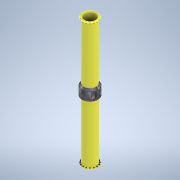
# Autodesk Inventor part: pipe_anode
Saved by Autodesk Inventor 2022 (Build 260153000, 153)
## iProperties
Created: 2021-12-16
Part Number: pipe_anode
Material: Steel
Document SubType Name: Modeling
Designer: jpc
Density: 7.85 g/cm^3
Appearance: Steel Galvanized
Mass: 2.14484e+06 g
Surface Area: 119776 cm^2
Volume: 273228 cm^3
Author: jpc
Autodesk Inventor part; units mm, degrees
ref_plane "XZ Plane" through (0, 0, 0) normal (0, 1, 0) x (-1, 0, 0)
ref_plane "XY Plane" through (0, 0, 0) normal (0, 0, 1) x (1, 0, 0)
sketch "cross_section" plane through (0, 0, 0) normal (0, 1, 0) x (-1, 0, 0)
  circle A0 centre (0, 0) radius 500
  circle A1 centre (0, 0) radius 450
  dimension "dia_out" = 1000
  dimension "dia_in" = 900
  constraints: 2 centre point, 2 coincident
  measures "dia_out" diameter of A0
  measures "dia_in" diameter of A1
sketch "curved_midline" plane through (0, 0, 0) normal (0, 0, 1) x (1, 0, 0)
  arc A0 (1000, 1000) -> (0, 0) centre (1000, 0) ccw
  line L0 (0, 0) -> (1000, 0) construction
  line L1 (1000, 0) -> (1000, 1000) construction
  dimension "d4" = 1000
  constraints: 4 end point, 2 point on circle, 1 centre point, 1 horizontal, 1 perpendicular
  measures "d4" distance of L0.end L1.end
sketch "straight_midline" plane through (0, 0, 0) normal (0, 0, 1) x (1, 0, 0)
  line L0 (0, 0) -> (0, 10000)
  dimension "len" = 10000
  constraints: 2 end point, 1 vertical
  measures "len" distance of L0.start L0.end
sweep "Sweep" add profiles "cross_section" path "straight_midline"
sketch "Sketch4" plane through (0, 0, 0) normal (0, -1, 0) x (1, 0, 0)
  circle A0 centre (0, 0) radius 600
  circle A1 centre (0, 0) radius 450 projected
  dimension "endcap_dia" = 1200
  constraints: 1 centre point, 1 coincident
  measures "endcap_dia" diameter of A0
extrude "Endcap" add sketch "Sketch4" against normal blind 50
ref_plane "Midplane" through (0, 5000, 0) normal (0, -1, 0) x (1, 0, 0)
chamfer "Chamfer" distance 12.5 angle 45 1 edges at (-600, 0, 0)
sketch "Sketch7" plane through (0, 50, 0) normal (0, 1, 0) x (1, 0, 0)
  circle A0 centre (0, 0) radius 600 construction
  circle A1 centre (0, 0) radius 600 construction
  line L0 (-600, 0) -> (-499.1664, 0) construction
  circle A2 centre (-549.5832, 0) radius 25.2084
  circle A3 centre (0, 0) radius 450 projected
  circle A4 centre (0, 0) radius 500 projected
  dimension "d27" = 100.8336
  dimension "d28" = 50.4168
  constraints: 2 end point, 1 centre point, 1 horizontal, 1 horizontal alignment, 1 midpoint, 1 other
  measures "d27" distance of L0.start L0.end
  measures "d28" diameter of A2
extrude "Hole" cut sketch "Sketch7" against normal through all contours A2
pattern_circular "Holes" count 16 over 360 about axis through (0, -10, 0) along (0, 1, 0) of "Hole"
mirror "MirroredFeatures" about plane through (0, 5000, 0) normal (0, -1, 0) of "Hole", "Holes", "Endcap", "Chamfer"
sketch "Sketch8" plane through (0, 50, 0) normal (0, 1, 0) x (1, 0, 0)
  circle A0 centre (-549.5832, 0) radius 25.2084 construction
  circle A1 centre (-549.5832, 0) radius 37.8126 construction
  circle A2 centre (0, 0) radius 587.5 construction
  line L0 (-587.5, 0) -> (-568.5416, 32.8369)
  line L1 (-568.5416, 32.8369) -> (-530.6248, 32.8369)
  line L2 (-530.6248, 32.8369) -> (-511.6664, 0)
  line L3 (-511.6664, 0) -> (-530.6248, -32.8369)
  line L4 (-530.6248, -32.8369) -> (-568.5416, -32.8369)
  line L5 (-568.5416, -32.8369) -> (-587.5, 0)
  dimension "d34" = 50.4168
  dimension "d35" = 75.6252
  constraints: 12 end point, 2 coincident, 1 centre point, 1 horizontal, 1 horizontal alignment, 14 other
  measures "d34" diameter of A0
  measures "d35" diameter of A1
extrude "BoltHead" add sketch "Sketch8" along normal blind 37.5 separate body
sketch "Sketch9" plane through (0, 50, 0) normal (0, -1, 0) x (1, 0, 0)
  circle A0 centre (-549.5832, 0) radius 25.2084 projected
  point P0 (0, 0)
extrude "BoltThreadHalf" add sketch "Sketch9" along normal blind 45 bodies 2
pattern_circular "BoltHalves" count 16 over 360 about axis through (0, -10, 0) along (0, 1, 0) bodies 2
mirror "MirroredBolts" about plane through (0, 5000, 0) normal (0, -1, 0) bodies 2
sketch "Sketch10" plane through (-530.6248, 9912.5, 32.8369) normal (0, -1, 0) x (0, 0, 1)
  circle A0 centre (-32.8369, 18.9584) radius 25.2084 projected
  point P0 (-32.8369, -530.6248)
extrude "ExtraThread" add sketch "Sketch10" along normal blind 22.5 bodies 2
chamfer "ThreadChamfer" distance 6.25 angle 45 1 edges at (-549.5832, 9890, -25.2084)
pattern_circular "Circular Pattern5" count 16 over 360 about axis through (0, 9950, 0) along (0, 1, 0) of "ExtraThread", "ThreadChamfer" bodies 2
sketch "Sketch11" plane through (0, 0, 0) normal (1, 0, 0) x (0, 1, 0)
  line L0 (10000, 450) -> (0, 450) construction
  line L1 (4491.6667, 450) -> (4666.6667, 625)
  line L2 (4666.6667, 625) -> (5333.3333, 625)
  line L3 (5333.3333, 625) -> (5508.3333, 450)
  line L4 (5508.3333, 450) -> (4491.6667, 450)
  line L5 (50, 500) -> (9950, 500) construction
  line L6 (-2000, 0) -> (12000, 0) projected
  point P0 (0, 0)
  point P1 (5000, 450)
  dimension "d54" = 666.6667
  dimension "d55" = 125
  dimension "d56" = 45
  constraints: 8 end point, 2 midpoint, 2 point on line, 1 collinear, 1 parallel, 1 perpendicular
  measures "d54" distance of L1.end L2.end
  measures "d55" distance between parallel lines of L2 L5
  measures "d56" angle of L0 L3
revolve "Attachment" add sketch "Sketch11" angle 360 about axis through (0, -10, 0) along (0, 1, 0) separate body
ref_plane "AnodeInnerPlane" through (450, 5000, 0) normal (1, 0, 0) x (0, 1, 0)
ref_plane "AnodOuterPlane" through (625, 5000, 0) normal (1, 0, 0) x (0, 1, 0)
ref_plane "NodeMidplane" through (537.5, 5000, 0) normal (1, 0, 0) x (0, 1, 0)
ref_plane "AnodeCutPlane" through (493.75, 5000, 0) normal (1, 0, 0) x (0, 1, 0)
split body "Split" result two bodies by plane through (0, 0, 0) normal (0, 0, 1) bodies 3 first body at (450.0712, 4830.5556, 19.6505)
sketch "Sketch13" plane through (0, 0, 0) normal (0, 1, 0) x (-1, 0, 0)
  line L0 (781.25, 15.625) -> (-781.25, 15.625)
  line L1 (-781.25, 15.625) -> (-781.25, -15.625)
  line L2 (-781.25, -15.625) -> (781.25, -15.625)
  line L3 (781.25, -15.625) -> (781.25, 15.625)
  arc A0 (-625, 0) -> (625, 0) centre (0, 0) ccw projected
  line L4 (625, 0) -> (450, 0) projected
  line L5 (781.25, 15.625) -> (-781.25, -15.625) construction
  dimension "d58" = 625
  dimension "d59" = 1562.5
  dimension "d60" = 31.25
  constraints: 10 end point, 2 parallel, 1 coincident, 1 horizontal, 1 midpoint, 1 perpendicular
  measures "d58" radius of A0
  measures "d59" distance of L1.end L2.end
  measures "d60" distance of L2.end L0.start
extrude "Separate" cut sketch "Sketch13" along normal through all both and the other way through all contours L3 L2 L1 L0 bodies 5 4
sketch "Sketch15" plane through (625, 5000, 0) normal (1, 0, 0) x (0, 1, 0)
  line L0 (-333.3333, 15.625) -> (333.3333, 15.625) construction
  line L1 (333.3333, 15.625) -> (333.3333, 15.625) construction
  line L2 (333.3333, 15.625) -> (-333.3333, 15.625) construction
  line L3 (-333.3333, 15.625) -> (-333.3333, 15.625) construction
  line L4 (333.3333, -15.625) -> (-333.3333, -15.625) construction
  line L5 (-333.3333, -15.625) -> (-333.3333, -15.625) construction
  line L6 (-333.3333, -15.625) -> (333.3333, -15.625) construction
  line L7 (333.3333, -15.625) -> (333.3333, -15.625) construction
  line L8 (333.3333, 15.625) -> (333.3333, 625) construction
  line L9 (-333.3333, 625) -> (333.3333, 625) construction
  line L10 (-333.3333, 15.625) -> (-333.3333, 625) construction
  line L11 (-333.3333, -625) -> (-333.3333, -15.625) construction
  line L12 (-333.3333, -625) -> (333.3333, -625) construction
  line L13 (333.3333, -625) -> (333.3333, -15.625) construction
  line L14 (250, 396.4844) -> (-250, 396.4844)
  line L15 (-250, 396.4844) -> (-250, 91.7969)
  line L16 (-250, 91.7969) -> (250, 91.7969)
  line L17 (250, 91.7969) -> (250, 396.4844)
  line L18 (250, -91.7969) -> (-250, -91.7969)
  line L19 (-250, -91.7969) -> (-250, -396.4844)
  line L20 (-250, -396.4844) -> (250, -396.4844)
  line L21 (250, -396.4844) -> (250, -91.7969)
  line L22 (0, 91.7969) -> (0, 15.625) construction
  point P0 (-5000, 0)
  dimension "d63" = 609.375
  dimension "d64" = 304.6875
  dimension "d65" = 666.6667
  dimension "d66" = 500
  dimension "d67" = 76.1719
  dimension "d68" = 76.1719
  constraints: 18 end point, 4 parallel, 3 perpendicular, 2 equal length, 2 horizontal, 2 midpoint, 1 collinear
  measures "d63" distance of L0.end L8.end
  measures "d64" distance of L16.end L14.start
  measures "d65" distance of L9.start L9.end
  measures "d66" distance of L14.start L14.end
  measures "d67" distance between parallel lines of L16 L0
  measures "d68" distance between parallel lines of L4 L18
extrude "BoltSurface" cut sketch "Sketch15" against normal up to surface (131.25 mm away) bodies 5 4
sketch "Sketch16" plane through (493.75, 5250, 91.7969) normal (0, 0, 1) x (1, 0, 0)
  line L0 (124.4719, 0) -> (124.4719, -500) construction
  line L1 (124.4719, 0) -> (0, 0) construction
  line L2 (0, 0) -> (0, -500) construction
  line L3 (124.4719, -500) -> (0, -500) construction
  line L4 (124.4719, 0) -> (0, 0) construction
  line L5 (62.236, 0) -> (62.236, -500) construction
  line L6 (124.4719, -500) -> (0, -500) construction
  circle A0 centre (62.236, -125) radius 31.118
  circle A1 centre (62.236, -375) radius 31.118
  point P0 (-493.75, -5250)
  dimension "d73" = 124.4719
  dimension "d74" = 500
  dimension "d75" = 125
  dimension "d76" = 125
  dimension "d77" = 62.236
  dimension "d78" = 62.236
  constraints: 2 centre point, 2 end point, 2 midpoint, 2 point on line
  measures "d73" distance of L0.start L1.end
  measures "d74" distance of L0.start L0.end
  measures "d75" distance from line of A0.centre L1
  measures "d76" distance from line of L3 A1.centre
  measures "d77" diameter of A0
  measures "d78" diameter of A1
extrude "BoltHoles" cut sketch "Sketch16" against normal through all bodies 4 5
mirror "Mirrored_Bolt_Hole_Cutouts" about plane through (0, 0, 0) normal (1, 0, 0) of "BoltHoles", "BoltSurface" bodies 5 4
sketch "Sketch17" plane through (493.75, 5250, 91.7969) normal (0, 0, 1) x (1, 0, 0)
  line L0 (124.4719, -500) -> (124.4719, 0) construction
  line L1 (124.4719, 0) -> (0, 0) construction
  line L2 (0, -500) -> (0, 0) construction
  circle A0 centre (62.236, -125) radius 31.118 construction
  circle A1 centre (62.236, -375) radius 31.118 construction
  line L3 (124.4719, -500) -> (0, -500) construction
  circle A2 centre (62.236, -375) radius 46.677 construction
  circle A3 centre (62.236, -125) radius 46.677 construction
  line L4 (38.8975, -84.5766) -> (85.5744, -84.5766)
  line L5 (85.5744, -84.5766) -> (108.9129, -125)
  line L6 (108.9129, -125) -> (85.5744, -165.4234)
  line L7 (85.5744, -165.4234) -> (38.8975, -165.4234)
  line L8 (38.8975, -165.4234) -> (15.559, -125)
  line L9 (15.559, -125) -> (38.8975, -84.5766)
  line L10 (102.6594, -351.6615) -> (102.6594, -398.3385)
  line L11 (102.6594, -398.3385) -> (62.236, -421.677)
  line L12 (62.236, -421.677) -> (21.8125, -398.3385)
  line L13 (21.8125, -398.3385) -> (21.8125, -351.6615)
  line L14 (21.8125, -351.6615) -> (62.236, -328.323)
  line L15 (62.236, -328.323) -> (102.6594, -351.6615)
  point P0 (-493.75, -5250)
  dimension "d82" = 93.3539
  dimension "d83" = 93.3539
  dimension "d81" = 62.236
  constraints: 24 end point, 4 coincident, 1 horizontal, 1 vertical, 32 other
  measures "d81" diameter of A0
extrude "anode_bolt_heads" add sketch "Sketch17" along normal blind 37.5 separate body
sketch "Sketch18" plane through (493.75, 5250, 91.7969) normal (0, 0, 1) x (1, 0, 0)
  circle A0 centre (62.236, -125) radius 31.118 projected
  circle A1 centre (62.236, -375) radius 31.118 projected
  point P0 (-493.75, -5250)
extrude "anode_bolt_threads" add sketch "Sketch18" against normal blind 262.5 bodies 6
chamfer "anode_bolt_thread_chamfers" distance 9.375 angle 45 2 edges at (524.868, 5125, -170.7031) (524.868, 4875, -170.7031)
mirror "anode_bolt_nuts" about plane through (0, 0, 0) normal (0, 0, 1) of "anode_bolt_heads" bodies 6
pattern_circular "Circular Pattern6" count 2 over 360 about axis through (0, -10, 0) along (0, 1, 0) of "anode_bolt_heads", "anode_bolt_threads", "anode_bolt_thread_chamfers", "anode_bolt_nuts" bodies 6
equation "\"d4\" = dia_out"
equation "\"endcap_dia\" = 1.2 * dia_out"
equation "\"endcap_thick\" = -0.5 * dia_in + 0.5 * dia_out"
equation "\"d28\" = 0.5 * d27"
equation "\"d35\" = 1.5 * d34"
equation "\"bolt_thick\" = 0.75 * endcap_thick"
equation "\"d38\" = 0.9 * endcap_thick"
equation "\"d43\" = 0.45 * endcap_thick"
equation "\"d48\" = 0.125 * endcap_thick"
equation "\"d54\" = 0.0666667 * len"
equation "\"d55\" = 0.125 * dia_out"
equation "\"d59\" = 2.5 * d58"
equation "\"d60\" = 0.05 * d58"
equation "\"d64\" = 0.5 * d63"
equation "\"d66\" = 0.75 * d65"
equation "\"d67\" = 0.25 * d64"
equation "\"d68\" = d67"
equation "\"d75\" = 0.25 * d74"
equation "\"d76\" = d75"
equation "\"d77\" = 0.5 * d73"
equation "\"d78\" = d77"
equation "\"d82\" = 1.5 * d81"
equation "\"d83\" = d82"
equation "\"d84\" = bolt_thick"
equation "\"d86\" = 7 * bolt_thick"
equation "\"d88\" = 0.25 * bolt_thick"
equation "\"d24\" = 0.25 * endcap_thick"
